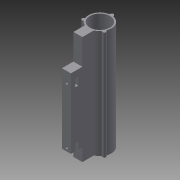
# Autodesk Inventor part: 知能ロボコンシリンダ２
Saved by Autodesk Inventor 2013 (Build 170138000, 138)
## iProperties
Created: 2014-05-28
Part Number: 知能ロボコンシリンダ２
Material: 一般
Document SubType Name: Modeling
Designer: horumo136
Density: 1 g/cm^3
Author: horumo136
Autodesk Inventor part; units mm, degrees
ref_plane "YZ Plane" through (0, 0, 0) normal (1, 0, 0) x (0, 1, 0)
ref_plane "XZ Plane" through (0, 0, 0) normal (0, 1, 0) x (-1, 0, 0)
ref_plane "XY Plane" through (0, 0, 0) normal (0, 0, 1) x (1, 0, 0)
sketch "スケッチ1" plane through (0, 0, 0) normal (0, 0, 1) x (1, 0, 0)
  circle A0 centre (0, 0) radius 11
  circle A1 centre (0, 0) radius 12.5
  dimension "d0" = 22
  dimension "d1" = 25
  constraints: 2 centre point, 2 coincident
  measures "d0" diameter of A0
  measures "d1" diameter of A1
extrude "押し出し1" add sketch "スケッチ1" along normal blind 100
sketch "スケッチ2" plane through (0, 0, 0) normal (0, 0, -1) x (-1, 0, 0)
  circle A0 centre (0, 0) radius 12.5 projected
extrude "押し出し2" add sketch "スケッチ2" along normal blind 3
sketch "スケッチ3" plane through (0, 0, 100) normal (0, 0, 1) x (1, 0, 0)
  circle A0 centre (0, 0) radius 12.5 projected
  line L0 (0, 12.5) -> (0, 14.9)
  line L1 (0, 12.5) -> (2.9783, 12.14)
  ellipse E0 centre (0, 12.5) end of major axis (1.9203, 12.5) minor radius 2.4
  circle A1 centre (0, 0) radius 11 projected
  ellipse E1 centre (-10.8253, -6.25) end of major axis (-11.7855, -4.587) minor radius 2.4
  ellipse E2 centre (10.8253, -6.25) end of major axis (9.8652, -7.913) minor radius 2.4
  point P0 (-12.9038, -7.45)
  point P1 (12.9038, -7.45)
  dimension "d6" = 2.4
  dimension "d7" = 3
  dimension "d12" = 360
  constraints: 4 end point, 3 coincident, 2 point on circle, 2 vertical, 1 vertical alignment, 22 other
  measures "d6" distance of L0.start L0.end
  measures "d7" distance of L0.start L1.end
extrude "押し出し4" add sketch "スケッチ3" against normal blind 103 contours E2 A0 | A0 E2 A1 | E0 L1 A0 | A0 L0 E0 | E0 A1 A0 L1 | A1 E2 | A0 E0 L0 | E0 A1 | E1 A0 | A0 E1 A1 | A1 E1 picked at (0.8508, 12.4175)
sketch "スケッチ4" plane through (0, 0, 100) normal (0, 0, 1) x (1, 0, 0)
  arc A0 (-9.739, -7.836) -> (9.739, -7.836) centre (0, 0) ccw projected
  circle A1 centre (0, 0) radius 11
  dimension "d16" = 22
  constraints: 2 coincident, 1 centre point
  measures "d16" diameter of A1
hole "穴1" at (0, 0, 100) direction (0, 0, -1) diameter 22 depth 100 tip angle 118
sketch "スケッチ5" plane through (0, 0, -3) normal (0, 0, -1) x (-1, 0, 0)
  arc A0 (-1.9166, 12.3522) -> (-11.6556, -4.5162) centre (0, 0) ccw projected
  circle A1 centre (0, 0) radius 12.5
  dimension "d54" = 0
  constraints: 1 centre point, 1 coincident
  measures "d54" radial gap between concentric circles of A0 A1
extrude "押し出し5" add sketch "スケッチ5" against normal blind 3
sketch "スケッチ6" plane through (0, 0, 100) normal (0, 0, 1) x (1, 0, 0)
  arc A0 (-9.739, -7.836) -> (9.739, -7.836) centre (0, 0) ccw projected
  line L0 (0, 0) -> (4.8841, -11.5063)
  line L1 (0, 0) -> (12.5, 0) construction
  line L2 (0, 0) -> (4.8841, -11.5063)
  line L3 (4.8841, -11.5063) -> (4.8841, -11.5063)
  line L4 (0, 0) -> (4.8841, -11.5063)
  line L5 (0, 0) -> (4.8841, -11.5063)
  line L6 (0, 0) -> (-4.8841, -11.5063)
  line L7 (0, 0) -> (12.5, 0) construction
  line L8 (-4.8841, -11.5063) -> (4.8841, -11.5063)
  arc A1 (-4.8841, -11.5063) -> (4.8841, -11.5063) centre (0, 0) ccw
  point P0 (0, -12.5)
  dimension "d26" = 67
  dimension "d27" = 113
  constraints: 18 end point, 7 point on circle, 2 collinear, 2 equal length, 2 horizontal, 1 centre point, 1 tangent
  measures "d26" angle of L0 L1
  measures "d27" angle of L6 L7
extrude "押し出し6" cut sketch "スケッチ6" against normal blind 103 contours L8 A0
sketch "スケッチ7" plane through (-4.8841, -11.5063, 100) normal (0, -1, 0) x (1, 0, 0)
  line L0 (0, 0) -> (9.7683, 0) projected
  line L1 (9.7683, 0) -> (9.7683, -103) projected
  line L2 (4.8841, 0) -> (4.8841, -24.5)
  line L3 (4.8841, -24.5) -> (4.8841, -85.5)
  line L4 (4.8841, -85.5) -> (4.8841, -90)
  point P0 (4.8841, -100)
  point P1 (9.7683, -100)
  dimension "d30" = 24.5
  dimension "d31" = 61
  dimension "d32" = 4.5
  constraints: 6 end point, 2 coincident, 1 collinear, 1 midpoint, 1 parallel, 1 point on line
  measures "d30" distance of L2.start L2.end
  measures "d31" distance of L2.end L3.end
  measures "d32" distance of L3.end L4.end
hole "穴2" at (0, -11.5063, 75.5) at (0, -11.5063, 14.5) direction (0, 1, 0) diameter 3 depth 8 tip angle 118
sketch "スケッチ10" plane through (0, 0, -3) normal (0, 0, -1) x (-1, 0, 0)
  line L0 (-4.8841, -11.5063) -> (4.8841, -11.5063)
  line L1 (4.8841, -11.5063) -> (4.8841, -36.5063)
  line L2 (4.8841, -36.5063) -> (-4.8841, -36.5063)
  line L3 (-4.8841, -36.5063) -> (-4.8841, -11.5063)
  dimension "d61" = 25
  constraints: 8 end point, 2 parallel, 1 horizontal, 1 perpendicular
  measures "d61" distance of L0.end L1.end
extrude "押し出し11" add sketch "スケッチ10" against normal blind 103
sketch "スケッチ11" plane through (-4.8841, -36.5063, -3) normal (0, -1, 0) x (1, 0, 0)
  line L0 (0, 103) -> (9.7683, 103) projected
  line L1 (0, 0) -> (0, 103) projected
  line L2 (4.8841, 103) -> (4.8841, 78.5)
  line L3 (4.8841, 78.5) -> (4.8841, 17.5)
  point P0 (4.8841, 3)
  dimension "d64" = 24.5
  dimension "d65" = 61
  constraints: 4 end point, 2 coincident, 1 collinear, 1 midpoint, 1 parallel
  measures "d64" distance of L2.start L2.end
  measures "d65" distance of L2.end L3.end
hole "穴4" at (0, -36.5063, 75.5) at (0, -36.5063, 14.5) direction (0, 1, 0) diameter 3 depth 24 tip angle 118
sketch "スケッチ13" plane through (4.8841, -36.5063, -3) normal (1, 0, 0) x (0, 0, -1)
  line L0 (0, 0) -> (-14, 0)
  line L1 (-14, 0) -> (-14, 12.5)
  line L2 (-14, 12.5) -> (0, 12.5)
  line L3 (0, 12.5) -> (0, 0)
  point P0 (-3, 36.5063)
  dimension "d77" = 14
  constraints: 8 end point, 2 parallel, 1 horizontal, 1 perpendicular
  measures "d77" distance of L1.end L2.end
extrude "押し出し13" cut sketch "スケッチ13" against normal blind 10
sketch "スケッチ14" plane through (4.8841, -36.5063, 100) normal (1, 0, 0) x (0, 0, -1)
  line L0 (0, 0) -> (0, 25) projected
  line L1 (89, 0) -> (89, 12.5) projected
  line L2 (89, 0) -> (89, 8)
  line L3 (89, 8) -> (0, 8)
  line L4 (89, 8) -> (81.5, 8)
  line L5 (81.5, 8) -> (81.5, 5)
  line L6 (81.5, 5) -> (89, 5)
  line L7 (89, 5) -> (89, 8)
  line L8 (0, 8) -> (0, 5)
  line L9 (0, 5) -> (22, 5)
  line L10 (22, 5) -> (28.5, 5)
  line L11 (28.5, 5) -> (28.5, 8)
  line L12 (22, 5) -> (20, 5)
  line L13 (20, 5) -> (20, 8)
  point P0 (100, 36.5063)
  dimension "d80" = 8
  dimension "d81" = 7.5
  dimension "d82" = 3
  dimension "d83" = 3
  dimension "d84" = 22
  dimension "d85" = 6.5
  dimension "d86" = 2
  constraints: 24 end point, 6 perpendicular, 6 point on line, 2 parallel, 1 horizontal
  measures "d80" distance of L1.start L2.end
  measures "d81" distance of L6.end L5.end
  measures "d82" distance of L5.end L4.end
  measures "d83" distance of L3.end L8.end
  measures "d84" distance of L8.end L9.end
  measures "d85" distance of L9.end L10.end
  measures "d86" distance of L9.end L12.end
extrude "押し出し14" cut sketch "スケッチ14" against normal blind 10 contours L13 L3 L11 L10 L9 | L6 L5 L3 L1
sketch "スケッチ16" plane through (0, 0, -3) normal (0, 0, -1) x (-1, 0, 0)
  line L0 (-4.8841, -24.0063) -> (4.8841, -24.0063) projected
  line L1 (4.8841, -24.0063) -> (4.8841, -11.5063) projected
  arc A0 (4.8841, -11.5063) -> (9.739, -7.836) centre (0, 0) ccw projected
  ellipse E0 centre (10.8253, -6.25) end of major axis (12.9038, -7.45) minor radius 1.9203 (9.739, -7.836) -> (11.6556, -4.5162) ccw projected
  arc A1 (11.6556, -4.5162) -> (1.9166, 12.3522) centre (0, 0) ccw projected
  ellipse E1 centre (0, 12.5) end of major axis (0, 14.9) minor radius 1.9203 (1.9166, 12.3522) -> (-1.9166, 12.3522) ccw projected
  arc A2 (-1.9166, 12.3522) -> (-11.6556, -4.5162) centre (0, 0) ccw projected
  ellipse E2 centre (-10.8253, -6.25) end of major axis (-12.9038, -7.45) minor radius 1.9203 (-11.6556, -4.5162) -> (-9.739, -7.836) ccw projected
  arc A3 (-9.739, -7.836) -> (-4.8841, -11.5063) centre (0, 0) ccw projected
  line L2 (-4.8841, -11.5063) -> (-4.8841, -24.0063) projected
  constraints: 3 other
sketch "スケッチ17" plane through (0, 0, 100) normal (0, 0, 1) x (1, 0, 0)
  arc A0 (4.8841, -11.5063) -> (9.739, -7.836) centre (0, 0) ccw projected
  ellipse E0 centre (10.8253, -6.25) end of major axis (12.9038, -7.45) minor radius 1.9203 (9.739, -7.836) -> (11.6556, -4.5162) ccw projected
  arc A1 (11.6556, -4.5162) -> (1.9166, 12.3522) centre (0, 0) ccw projected
  ellipse E1 centre (0, 12.5) end of major axis (0, 14.9) minor radius 1.9203 (1.9166, 12.3522) -> (-1.9166, 12.3522) ccw projected
  arc A2 (-1.9166, 12.3522) -> (-11.6556, -4.5162) centre (0, 0) ccw projected
  ellipse E2 centre (-10.8253, -6.25) end of major axis (-12.9038, -7.45) minor radius 1.9203 (-11.6556, -4.5162) -> (-9.739, -7.836) ccw projected
  arc A3 (-9.739, -7.836) -> (-4.8841, -11.5063) centre (0, 0) ccw projected
  line L0 (-4.8841, -11.5063) -> (-4.8841, -36.5063) projected
  line L1 (-4.8841, -36.5063) -> (4.8841, -36.5063) projected
  line L2 (4.8841, -36.5063) -> (4.8841, -11.5063) projected
  circle A4 centre (0, 0) radius 11 projected
  constraints: 3 other
extrude "押し出し15" add sketch "スケッチ17" along normal blind 10
sketch "スケッチ18" plane through (-4.8841, -24.0063, -3) normal (-1, 0, 0) x (0, 0, 1)
  line L0 (113, -12.5) -> (90, -12.5)
  line L1 (90, -12.5) -> (90, 0)
  line L2 (90, 0) -> (113, 0)
  line L3 (113, 0) -> (113, -12.5)
  point P0 (3, 24.0063)
  dimension "d91" = 23
  constraints: 8 end point, 2 parallel, 1 horizontal, 1 perpendicular
  measures "d91" distance of L1.end L2.end
extrude "押し出し16" cut sketch "スケッチ18" against normal blind 10
sketch "スケッチ19" plane through (0, 0, 110) normal (0, 0, 1) x (1, 0, 0)
  line L0 (-4.8841, -24.0063) -> (4.8841, -24.0063) projected
  line L1 (4.8841, -24.0063) -> (4.8841, -11.5063) projected
  arc A0 (4.8841, -11.5063) -> (9.739, -7.836) centre (0, 0) ccw projected
  ellipse E0 centre (10.8253, -6.25) end of major axis (12.9038, -7.45) minor radius 1.9203 (9.739, -7.836) -> (11.6556, -4.5162) ccw projected
  arc A1 (11.6556, -4.5162) -> (1.9166, 12.3522) centre (0, 0) ccw projected
  ellipse E1 centre (0, 12.5) end of major axis (0, 14.9) minor radius 1.9203 (1.9166, 12.3522) -> (-1.9166, 12.3522) ccw projected
  arc A2 (-1.9166, 12.3522) -> (-11.6556, -4.5162) centre (0, 0) ccw projected
  ellipse E2 centre (-10.8253, -6.25) end of major axis (-12.9038, -7.45) minor radius 1.9203 (-11.6556, -4.5162) -> (-9.739, -7.836) ccw projected
  arc A3 (-9.739, -7.836) -> (-4.8841, -11.5063) centre (0, 0) ccw projected
  line L2 (-4.8841, -11.5063) -> (-4.8841, -24.0063) projected
  circle A4 centre (0, 0) radius 11 projected
  constraints: 3 other
extrude "押し出し17" add sketch "スケッチ19" along normal blind 5
